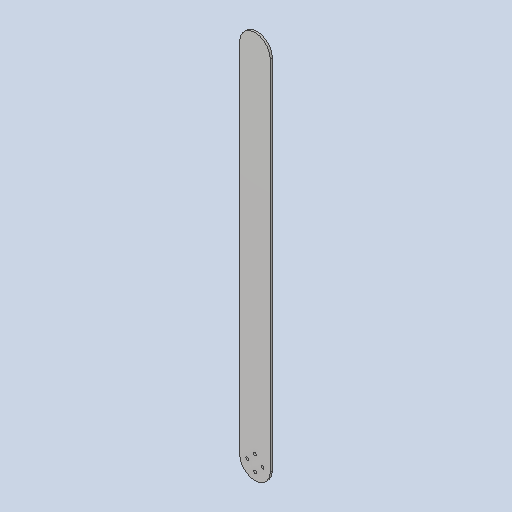
# Autodesk Inventor part: arm_link
Saved by Autodesk Inventor 2022 (Build 260153000, 153)
## iProperties
Category: リンク
Created: 2016-08-23
Part Number: arm_link
Material: GFRP
Document SubType Name: Modeling
Designer: hiro
Density: 1.75 g/cm^3
Appearance: 滑らか - 淡い灰色
Mass: 6.98824 g
Surface Area: 46.6416 cm^2
Volume: 3.99328 cm^3
Author: hiro
Autodesk Inventor part; units mm, degrees
ref_plane "YZ Plane" through (0, 0, 0) normal (1, 0, 0) x (0, 1, 0)
ref_plane "XZ Plane" through (0, 0, 0) normal (0, 1, 0) x (-1, 0, 0)
ref_plane "XY Plane" through (0, 0, 0) normal (0, 0, 1) x (1, 0, 0)
sketch "スケッチ1" plane through (0, 0, 0) normal (0, 0, 1) x (1, 0, 0)
  line L0 (30, 0) -> (30, 350)
  line L1 (0, 350) -> (0, 0)
  arc A0 (30, 350) -> (0, 350) centre (15, 350) ccw
  arc A1 (0, 0) -> (30, 0) centre (15, 0) ccw
  dimension "d35" = 30
  dimension "d36" = 350
  constraints: 4 end point, 4 point on circle, 3 horizontal alignment, 2 centre point, 1 parallel
  measures "d35" distance of L0.start L1.end
  measures "d36" distance of L1.start L1.end
extrude "押し出し1" add sketch "スケッチ1" along normal blind 2
sketch "スケッチ3" plane through (0, 0, 2) normal (0, 0, 1) x (1, 0, 0)
  line L0 (0, 350) -> (0, 0) projected
  arc A0 (0, 0) -> (30, 0) centre (15, 0) ccw projected
  line L1 (0, 0) -> (30, 0) construction
  point P0 (7.5, 0)
  point P1 (15, -7.5)
  point P2 (22.5, 0)
  point P3 (15, 7.5)
  dimension "d41" = 7.5
  dimension "d44" = 360
  constraints: 2 end point, 1 horizontal, 1 point on line, 5 other
  measures "d41" distance of point (7.5, 0) A0.centre
hole "穴1" at (7.5, 0, 2) at (15, -7.5, 2) at (22.5, 0, 2) at (15, 7.5, 2) direction (0, 0, -1) diameter 2.8 end through all
